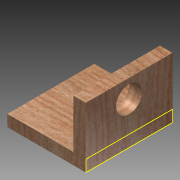
# Autodesk Inventor part: Pulling Bracket
Saved by Autodesk Inventor 2014 SP1 (Build 180222100, 222)
## iProperties
Created: 2014-11-20
Part Number: Pulling Bracket
Material: Generic
Document SubType Name: Modeling
Designer: AlecShufelt
Density: 1 g/cm^3
Appearance: Birch - Natural Polished
Author: AlecShufelt
Autodesk Inventor part; units mm, degrees
ref_plane "YZ Plane" through (0, 0, 0) normal (1, 0, 0) x (0, 1, 0)
ref_plane "XZ Plane" through (0, 0, 0) normal (0, 1, 0) x (-1, 0, 0)
ref_plane "XY Plane" through (0, 0, 0) normal (0, 0, 1) x (1, 0, 0)
sketch "Sketch1" plane through (0, 0, 0) normal (0, 1, 0) x (-1, 0, 0)
  line L0 (0, 0) -> (-136.5758, 0)
  line L1 (-136.5758, 0) -> (-136.5758, 151.384)
  line L2 (-136.5758, 151.384) -> (0, 151.384)
  line L3 (0, 151.384) -> (0, 0)
  dimension "d0" = 136.5758
  dimension "d1" = 151.384
  constraints: 8 end point, 2 parallel, 1 horizontal, 1 perpendicular
  measures "d0" distance of L1.end L2.end
  measures "d1" distance of L0.end L1.end
extrude "Extrusion1" add sketch "Sketch1" along normal blind 20.1676
sketch "Sketch2" plane through (136.5758, 0, 151.384) normal (1, 0, 0) x (0, 0, -1)
  line L0 (151.384, 0) -> (0, 0) projected
  line L1 (151.384, 0) -> (151.384, 20.1676) projected
  line L2 (0, 20.1676) -> (151.384, 20.1676) projected
  line L3 (0, 0) -> (0, 20.1676) projected
sketch "Sketch3" plane through (0, 20.1676, 0) normal (0, 1, 0) x (1, 0, 0)
  line L0 (0, -151.384) -> (136.5758, -151.384) projected
  line L1 (136.5758, 0) -> (114.7572, 0)
  line L2 (114.7572, 0) -> (114.7572, -151.384)
  line L3 (114.7572, -151.384) -> (136.5758, -151.384)
  line L4 (136.5758, -151.384) -> (136.5758, 0)
  dimension "d4" = 21.8186
  constraints: 8 end point, 2 parallel, 1 horizontal, 1 perpendicular, 1 point on line
  measures "d4" distance of L3.end L2.end
extrude "Extrusion2" add sketch "Sketch3" along normal blind 84.8614
sketch "Sketch4" plane through (136.5758, 0, 151.384) normal (1, 0, 0) x (0, 0, -1)
  line L0 (0, 105.029) -> (151.384, 105.029) projected
  circle A0 centre (75.692, 72.9361) radius 22.6695
  dimension "d7" = 45.339
  dimension "d8" = 32.0929
  constraints: 1 centre point
  measures "d7" diameter of A0
  measures "d8" distance from line of L0 A0.centre
extrude "Extrusion3" cut sketch "Sketch4" against normal blind 84.8614
body "Solid1"
